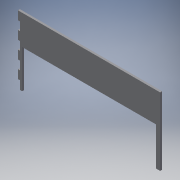
# Autodesk Inventor part: PCBWall
Saved by Autodesk Inventor 2017 (Build 210142000, 142)
## iProperties
Created: 2017-03-28
Part Number: PCBWall
Material: Generic
Document SubType Name: Modeling
Designer: hoeflinc
Density: 1 g/cm^3
Appearance: Default
Quantity: 1
Author: hoeflinc
Autodesk Inventor part; units mm, degrees
ref_plane "YZ Plane" through (0, 0, 0) normal (1, 0, 0) x (0, 1, 0)
ref_plane "XZ Plane" through (0, 0, 0) normal (0, 1, 0) x (-1, 0, 0)
ref_plane "XY Plane" through (0, 0, 0) normal (0, 0, 1) x (1, 0, 0)
sketch "Sketch1" plane through (0, 0, 0) normal (0, 0, 1) x (1, 0, 0)
  line L0 (0, 0) -> (212.725, 0)
  line L1 (212.725, 0) -> (212.725, 101.6)
  line L2 (212.725, 101.6) -> (0, 101.6)
  line L3 (0, 101.6) -> (0, 0)
  dimension "d0" = 212.725
  dimension "d1" = 101.6
  constraints: 8 end point, 2 parallel, 1 horizontal, 1 perpendicular
  measures "d0" distance of L1.end L2.end
  measures "d1" distance of L2.end L0.start
extrude "Extrusion1" add sketch "Sketch1" along normal blind 3
sketch "Sketch2" plane through (0, 0, 3) normal (0, 0, 1) x (1, 0, 0)
  line L0 (6.35, 0) -> (206.375, 0)
  line L1 (206.375, 0) -> (206.375, 57.15)
  line L2 (206.375, 57.15) -> (6.35, 57.15)
  line L3 (6.35, 57.15) -> (6.35, 0)
  line L4 (0, 0) -> (212.725, 0) projected
  line L5 (212.725, 0) -> (212.725, 101.6) projected
  line L6 (212.725, 101.6) -> (0, 101.6) projected
  line L7 (0, 101.6) -> (0, 0) projected
  dimension "d4" = 57.15
  dimension "d9" = 6.35
  dimension "d10" = 6.35
  constraints: 8 end point, 2 parallel, 1 horizontal, 1 perpendicular
  measures "d4" distance of L2.end L0.start
  measures "d9" distance between parallel lines of L5 L1
  measures "d10" distance between parallel lines of L7 L3
extrude "Extrusion2" cut sketch "Sketch2" against normal blind 3.5 contours L3 L2 L1 L0
sketch "Sketch3" plane through (0, 0, 3) normal (0, 0, 1) x (1, 0, 0)
  line L0 (206.375, 57.15) -> (206.375, 0) projected
  line L1 (206.375, 0) -> (212.725, 0) projected
  line L2 (212.725, 0) -> (212.725, 101.6) projected
  line L3 (212.725, 101.6) -> (0, 101.6) projected
  line L4 (0, 101.6) -> (0, 0) projected
  line L5 (0, 0) -> (6.35, 0) projected
  line L6 (6.35, 0) -> (6.35, 57.15) projected
  line L7 (6.35, 57.15) -> (206.375, 57.15) projected
  line L8 (0, 0) -> (3, 0)
  line L9 (3, 0) -> (3, 12.5984)
  line L10 (3, 12.5984) -> (0, 12.5984)
  line L11 (0, 12.5984) -> (0, 0)
  line L12 (3, 25.4) -> (3, 37.9984)
  line L13 (3, 37.9984) -> (0, 37.9984)
  line L14 (0, 37.9984) -> (0, 25.4)
  line L15 (0, 25.4) -> (3, 25.4)
  line L16 (3, 50.8) -> (3, 63.3984)
  line L17 (3, 63.3984) -> (0, 63.3984)
  line L18 (0, 63.3984) -> (0, 50.8)
  line L19 (0, 50.8) -> (3, 50.8)
  line L20 (3, 76.2) -> (3, 88.7984)
  line L21 (3, 88.7984) -> (0, 88.7984)
  line L22 (0, 88.7984) -> (0, 76.2)
  line L23 (0, 76.2) -> (3, 76.2)
  line L24 (3, 101.6) -> (3, 114.1984)
  line L25 (3, 114.1984) -> (0, 114.1984)
  line L26 (0, 114.1984) -> (0, 101.6)
  line L27 (0, 101.6) -> (3, 101.6)
  dimension "d11" = 12.5984
  dimension "d12" = 3
  dimension "d15" = 25.4
  constraints: 40 end point, 2 parallel, 1 horizontal, 1 perpendicular, 1 vertical, 32 other
  measures "d11" distance of L8.end L9.end
  measures "d12" distance between parallel lines of L4 L9
  measures "d15" distance of L8.end L12.start
extrude "Extrusion3" cut sketch "Sketch3" against normal blind 3 contours L5 L4 L10 L9 | L3 L26 L25 L24 | L21 L20 L23 L4 | L4 L13 L12 L15 | L17 L16 L19 L4
body "Solid1"
